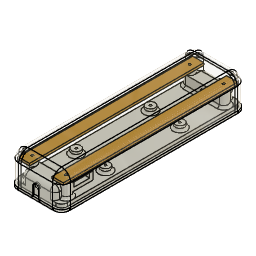
MQTT_Lamp (Autodesk Fusion 360 design; units mm, degrees)
Autodesk Fusion 360 part; units mm, degrees
sketch "Sketch1" plane through (0, 0, 0) normal (0, 0, 1) x (1, 0, 0) in component "base"
  line L0 (0, 0) -> (42, 0)
  line L1 (42, 0) -> (42, 160)
  line L2 (42, 160) -> (0, 160)
  line L3 (0, 160) -> (0, 0)
  dimension "d1" = 42
  dimension "d2" = 160
  constraint horizontal L0
  constraint vertical L1
  constraint horizontal L2
  constraint vertical L3
  constraint coincident L0.start L3.end
  measures "d1" distance of L0.start L0.end
  measures "d2" distance of L0.start L2.end
extrude "Extrude1" add sketch "Sketch1" along normal blind 5 makes body 1 in component "base"
sketch "Sketch2" plane through (0, 0, 5) normal (0, 0, 1) x (-1, 0, 0) in component "base"
  line L0 (0, -160) -> (0, 0)
  line L1 (0, 0) -> (-42, 0)
  line L2 (-42, 0) -> (-42, -160)
  line L3 (-42, -160) -> (0, -160)
  line L4 (-21, -160) -> (-21, 0)
  line L5 (-36, -150) -> (-6, -150)
  line L6 (-6, -150) -> (-6, -10)
  line L7 (-6, -10) -> (-36, -10)
  line L8 (-36, -10) -> (-36, -150)
  line L9 (-36, -150) -> (-6, -10) construction
  line L10 (-6, -150) -> (-36, -10) construction
  circle A0 centre (-6, -150) radius 1
  circle A1 centre (-36, -150) radius 1
  circle A2 centre (-6, -10) radius 1
  circle A3 centre (-36, -10) radius 1
  circle A4 centre (-36, -150) radius 4
  circle A5 centre (-6, -150) radius 4
  circle A6 centre (-6, -10) radius 4
  circle A7 centre (-36, -10) radius 4
  point P0 (-21, -80)
  dimension "d5" = 30
  dimension "d6" = 140
  dimension "d7" = 2
  dimension "d8" = 2
  dimension "d9" = 2
  dimension "d10" = 2
  dimension "d11" = 3
  dimension "d12" = 3
  dimension "d13" = 3
  dimension "d14" = 3
  constraint midpoint L3 L4.start
  constraint midpoint L1 L4.end
  constraint horizontal L5
  constraint perpendicular L5 L6
  constraint parallel L5 L7
  constraint parallel L6 L8
  constraint coincident L9 P0
  constraint coincident L10 P0
  constraint midpoint L4 P0
  constraint coincident L5.end L6.start
  constraint coincident L5.start L8.end
  constraint coincident L6.end L7.start
  constraint coincident L7.end L8.start
  measures "d5" distance of L6.end L7.end
  measures "d6" distance of L5.end L6.end
  measures "d7" diameter of A0
  measures "d8" diameter of A1
  measures "d9" diameter of A2
  measures "d10" diameter of A3
extrude "Extrude2" add sketch "Sketch2" along normal blind 14 contours L5 L8 A1 A4 | L5 L8 A1 A4 | L5 L6 A0 A5 | L5 L6 A0 A5 | L6 L7 A2 A6 | L6 L7 A2 A6 | L7 L8 A3 A7 | L7 L8 A3 A7 bodies 1 in component "base"
sketch "Sketch3" plane through (0, 0, 5) normal (0, 0, 1) x (-1, 0, 0) in component "base"
  circle A0 centre (-6, -150) radius 4
  circle A1 centre (-36, -150) radius 4
  line L0 (0, -160) -> (0, 0)
  line L1 (0, 0) -> (-42, 0)
  line L2 (-42, 0) -> (-42, -160)
  line L3 (-42, -160) -> (0, -160)
  circle A2 centre (-36, -10) radius 4
  circle A3 centre (-6, -10) radius 4
  line L4 (-6, -10) -> (-6, 0)
  line L5 (-6, 0) -> (-36, 0)
  line L6 (-36, 0) -> (-36, -14)
  line L7 (-36, -14) -> (-6, -14)
  line L8 (-6, -14) -> (-6, 0)
  line L9 (-36, -150) -> (-36, -160)
  line L10 (-36, -160) -> (-6, -160)
  line L11 (-6, -160) -> (-6, -146)
  line L12 (-6, -146) -> (-36, -146)
  line L13 (-36, -146) -> (-36, -160)
  constraint coincident A3.centre L4.start
  constraint coincident L1 L4.end
  constraint perpendicular L1 L4
  constraint horizontal L5
  constraint vertical L6
  constraint horizontal L7
  constraint vertical L8
  constraint coincident A2 L6.end
  constraint coincident A1.centre L9.start
  constraint coincident L3 L9.end
  constraint perpendicular L3 L9
  constraint horizontal L10
  constraint vertical L11
  constraint horizontal L12
  constraint vertical L13
  constraint coincident A0 L11.end
extrude "Extrude3" add sketch "Sketch3" along normal blind 10 contours A0 A1 L3 L9 L10 L11 L12 L13 | L1 A2 A3 L4 L5 L6 L7 L8 bodies 1 in component "base"
sketch "Sketch4" plane through (0, 0, 0) normal (0, -1, 0) x (1, 0, 0) in component "base"
  line L0 (0, 0) -> (42, 0)
  line L1 (42, 0) -> (42, 5)
  line L2 (42, 5) -> (36, 5)
  line L3 (36, 5) -> (36, 15)
  line L4 (36, 15) -> (6, 15)
  line L5 (6, 15) -> (6, 5)
  line L6 (6, 5) -> (0, 5)
  line L7 (0, 5) -> (0, 0)
  line L8 (6, 5) -> (36, 5)
  line L9 (21, 5) -> (21, 15)
  circle A0 centre (21, 10) radius 2.5
  dimension "d19" = 5
  constraint coincident L5.end L6.start
  constraint coincident L2.end L3.start
  constraint midpoint L8 L9.start
  constraint midpoint L4 L9.end
  constraint midpoint L9 A0.centre
  measures "d19" diameter of A0
extrude "Extrude4" cut sketch "Sketch4" against normal blind 14 contours L9 A0 | L9 A0 bodies 1 in component "base"
sketch "Sketch5" plane through (0, 160, 0) normal (0, 1, 0) x (-1, 0, 0) in component "base"
  line L0 (-42, 0) -> (0, 0)
  line L1 (0, 0) -> (0, 5)
  line L2 (0, 5) -> (-6, 5)
  line L3 (-6, 5) -> (-6, 15)
  line L4 (-6, 15) -> (-36, 15)
  line L5 (-36, 15) -> (-36, 5)
  line L6 (-36, 5) -> (-42, 5)
  line L7 (-42, 5) -> (-42, 0)
  line L8 (-36, 5) -> (-6, 5)
  line L9 (-21, 5) -> (-21, 15)
  circle A0 centre (-21, 10) radius 1.5
  dimension "d22" = 3
  constraint coincident L5.end L6.start
  constraint coincident L2.end L3.start
  constraint midpoint L8 L9.start
  constraint midpoint L4 L9.end
  constraint midpoint L9 A0.centre
  measures "d22" diameter of A0
extrude "Extrude5" cut sketch "Sketch5" against normal blind 14 contours L9 A0 | L9 A0 bodies 1 in component "base"
sketch "Sketch6" plane through (0, 0, 5) normal (0, 0, 1) x (-1, 0, 0) in component "base"
  line L0 (-6, -14) -> (-36, -14)
  arc A0 (-36, -6) -> (-36, -14) centre (-36, -10) ccw
  line L1 (-36, -6) -> (-36, 0)
  line L2 (-36, 0) -> (-42, 0)
  line L3 (-42, 0) -> (-42, -160)
  line L4 (-42, -160) -> (-36, -160)
  line L5 (-36, -160) -> (-36, -154)
  arc A1 (-36, -146) -> (-36, -154) centre (-36, -150) ccw
  line L6 (-36, -146) -> (-6, -146)
  arc A2 (-6, -154) -> (-6, -146) centre (-6, -150) ccw
  line L7 (-6, -154) -> (-6, -160)
  line L8 (-6, -160) -> (0, -160)
  line L9 (0, -160) -> (0, 0)
  line L10 (0, 0) -> (-6, 0)
  line L11 (-6, 0) -> (-6, -6)
  arc A3 (-6, -14) -> (-6, -6) centre (-6, -10) ccw
  line L12 (-36, -14) -> (-28, -14)
  line L13 (-28, -14) -> (-28, -34)
  line L14 (-28, -34) -> (-36, -34)
  line L15 (-36, -34) -> (-36, -14)
  dimension "d25" = 8
  dimension "d26" = 20
  constraint horizontal L12
  constraint vertical L13
  constraint horizontal L14
  constraint vertical L15
  constraint coincident L0.end A0.end
  measures "d25" distance of L0.end L12.end
  measures "d26" distance of L0.end L14.end
extrude "Extrude6" add sketch "Sketch6" along normal blind 10 contours L0 L12 L13 L14 L15 bodies 1 in component "base"
sketch "Sketch7" plane through (28, 0, 0) normal (-1, 0, 0) x (0, -1, 0) in component "base"
  line L0 (-34, 5) -> (-14, 5)
  line L1 (-14, 5) -> (-14, 15)
  line L2 (-14, 15) -> (-34, 15)
  line L3 (-34, 15) -> (-34, 5)
  line L4 (-31, 8) -> (-17, 8)
  line L5 (-17, 8) -> (-17, 12)
  line L6 (-17, 12) -> (-31, 12)
  line L7 (-31, 12) -> (-31, 8)
  dimension "d29" = -3
extrude "Extrude7" cut sketch "Sketch7" against normal blind 8 contours L4 L5 L6 L7 bodies 1 in component "base"
fillet "Fillet1" radius 3 2 edges at (28, 24, 15) (36, 24, 15) on bodies 1 in component "base"
fillet "Fillet2" radius 3 2 edges at (28.8787, 14, 14.1213) (28, 14, 8.5) on bodies 1 in component "base"
fillet "Fillet3" radius 5 4 edges at (42, 0, 2.5) (0, 0, 2.5) (42, 160, 2.5) (0, 160, 2.5) on bodies 1 in component "base"
fillet "Fillet4" radius 2 8 edges at (40, 150, 5) (21, 146, 5) (2, 150, 5) (40, 10, 5) (2, 10, 5) (15.5, 14, 5) (27.1213, 14.8787, 5) (28, 25.5, 5) on bodies 1 in component "base"
fillet "Fillet5" radius 4 10 edges at (6, 3, 15) (6, 0, 10) (21, 0, 15) (36, 0, 10) (36, 3, 15) (21, 160, 15) (36, 157, 15) (36, 160, 10) (6, 157, 15) (6, 160, 10) on bodies 1 in component "base"
sketch "Sketch9" plane through (0, 0, 5) normal (0, 0, 1) x (-1, 0, 0) in component "base"
  line L0 (-26, -34) -> (-36, -34)
  line L1 (-36, -34) -> (-36, -16)
  arc A0 (-42, -10) -> (-36, -16) centre (-36, -10) ccw
  line L2 (-42, -10) -> (-42, -150)
  arc A1 (-36, -144) -> (-42, -150) centre (-36, -150) ccw
  line L3 (-36, -144) -> (-6, -144)
  arc A2 (0, -150) -> (-6, -144) centre (-6, -150) ccw
  line L4 (0, -150) -> (0, -10)
  arc A3 (-6, -16) -> (0, -10) centre (-6, -10) ccw
  line L5 (-6, -16) -> (-25, -16)
  arc A4 (-25, -16) -> (-26, -17) centre (-25, -17) ccw
  line L6 (-26, -17) -> (-26, -34)
  line L7 (-42, -80) -> (0, -80)
  line L8 (-34, -113) -> (-8, -113)
  line L9 (-8, -113) -> (-8, -47)
  line L10 (-8, -47) -> (-34, -47)
  line L11 (-34, -47) -> (-34, -113)
  line L12 (-34, -113) -> (-8, -47) construction
  line L13 (-8, -113) -> (-34, -47) construction
  circle A5 centre (-8, -47) radius 1
  circle A6 centre (-34, -47) radius 1
  circle A7 centre (-8, -113) radius 1
  circle A8 centre (-34, -113) radius 1
  circle A9 centre (-34, -113) radius 4
  circle A10 centre (-8, -113) radius 4
  circle A11 centre (-8, -47) radius 4
  circle A12 centre (-34, -47) radius 4
  point P0 (-21, -80)
  dimension "d48" = 26
  dimension "d49" = 66
  dimension "d50" = 2
  dimension "d51" = 2
  dimension "d52" = 2
  dimension "d53" = 2
  dimension "d54" = 3
  dimension "d55" = 3
  dimension "d56" = 3
  dimension "d57" = 3
  constraint midpoint L2 L7.start
  constraint midpoint L4 L7.end
  constraint horizontal L8
  constraint perpendicular L8 L9
  constraint parallel L8 L10
  constraint parallel L9 L11
  constraint coincident L12 P0
  constraint coincident L13 P0
  constraint midpoint L7 P0
  constraint coincident L9.end L10.start
  constraint coincident L10.end L11.start
  constraint coincident L8.end L9.start
  constraint coincident L8.start L11.end
  measures "d48" distance of L9.end L10.end
  measures "d49" distance of L8.end L9.end
  measures "d50" diameter of A5
  measures "d51" diameter of A6
  measures "d52" diameter of A7
  measures "d53" diameter of A8
extrude "Extrude9" add sketch "Sketch9" along normal blind 4 contours L10 L11 A6 A12 | L10 L11 A6 A12 | L8 L11 A8 A9 | L8 L11 A8 A9 | L8 L9 A7 A10 | L8 L9 A7 A10 | L9 L10 A5 A11 | L9 L10 A5 A11 bodies 1 in component "base"
sketch "Sketch1 (2)" plane through (0, 0, 19) normal (0, 0, 1) x (-1, 0, 0) in component "light"
  circle A0 centre (-6, -10) radius 1
  circle A1 centre (-6, -10) radius 4
sketch "Sketch2 (2)" plane through (0, 0, 0) normal (0, 0, 1) x (1, 0, 0) in component "light"
  line L0 (0, 0) -> (10, 0)
  line L1 (10, 0) -> (10, 155)
  line L2 (10, 155) -> (0, 155)
  line L3 (0, 155) -> (0, 0)
  line L4 (5, 155) -> (5, 0)
  line L5 (5, 77.5) -> (5, 147.5)
  line L6 (5, 77.5) -> (5, 7.5)
  circle A0 centre (5, 7.5) radius 1
  circle A1 centre (5, 147.5) radius 1
  dimension "d62" = 10
  dimension "d63" = 155
  dimension "d64" = 70
  dimension "d65" = 70
  dimension "d66" = 2
  dimension "d67" = 2
  constraint horizontal L0
  constraint vertical L1
  constraint horizontal L2
  constraint vertical L3
  constraint coincident L0.start L3.end
  constraint midpoint L2 L4.start
  constraint midpoint L0 L4.end
  constraint midpoint L4 L5.start
  constraint perpendicular L0 L5
  constraint parallel L4 L6
  constraint coincident L6.end A0.centre
  constraint coincident L5.end A1.centre
  measures "d62" distance of L0.start L0.end
  measures "d63" distance of L0.start L2.end
  measures "d64" distance of L5.start L5.end
  measures "d65" distance of L5.start L6.end
  measures "d66" diameter of A0
  measures "d67" diameter of A1
extrude "Extrude1'" add sketch "Sketch2 (2)" along normal blind 2 separate body contours L0 L2 L3 L4 L5 L6 A0 A1 | L0 L1 L2 L4 L5 L6 A0 A1 makes body 2 in component "light"
move_body "Move1" bodies 2 to x (1, 0, 0) y (0, 1, 0) z (0, 0, 1) at (1, 2.5, 19) in component "light"
sketch "Sketch1 (3)" plane through (0, 0, 0) normal (0, 0, -1) x (1, 0, 0)
  arc A0 (0, -155) -> (5, -160) centre (5, -155) ccw
  line L0 (5, -160) -> (37, -160)
  arc A1 (37, -160) -> (42, -155) centre (37, -155) ccw
  line L1 (42, -155) -> (42, -5)
  arc A2 (42, -5) -> (37, 0) centre (37, -5) ccw
  line L2 (37, 0) -> (5, 0)
  arc A3 (5, 0) -> (0, -5) centre (5, -5) ccw
  line L3 (0, -5) -> (0, -155)
  line L4 (37, 2) -> (5, 2)
  arc A4 (5, 2) -> (-2, -5) centre (5, -5) ccw
  line L5 (-2, -5) -> (-2, -155)
  arc A5 (-2, -155) -> (5, -162) centre (5, -155) ccw
  line L6 (5, -162) -> (37, -162)
  arc A6 (37, -162) -> (44, -155) centre (37, -155) ccw
  line L7 (44, -155) -> (44, -5)
  arc A7 (44, -5) -> (37, 2) centre (37, -5) ccw
  dimension "d70" = 2
extrude "Extrude10" add sketch "Sketch1 (3)" against normal blind 2 bodies 1 in component "base"
sketch "Sketch2 (3)" plane through (0, 0, 5) normal (0, 0, 1) x (-1, 0, 0)
  line L0 (-26, -34) -> (-36, -34)
  line L1 (-36, -34) -> (-36, -16)
  arc A0 (-42, -10) -> (-36, -16) centre (-36, -10) ccw
  line L2 (-42, -10) -> (-42, -150)
  arc A1 (-36, -144) -> (-42, -150) centre (-36, -150) ccw
  line L3 (-36, -144) -> (-6, -144)
  arc A2 (0, -150) -> (-6, -144) centre (-6, -150) ccw
  line L4 (0, -150) -> (0, -10)
  arc A3 (-6, -16) -> (0, -10) centre (-6, -10) ccw
  line L5 (-6, -16) -> (-25, -16)
  arc A4 (-25, -16) -> (-26, -17) centre (-25, -17) ccw
  line L6 (-26, -17) -> (-26, -34)
  line L7 (-21, -144) -> (-21, -16)
  line L8 (-21, -80) -> (-21, -130)
  line L9 (-21, -80) -> (-21, -30)
  circle A5 centre (-21, -30) radius 2
  circle A6 centre (-21, -130) radius 2
  circle A7 centre (-8, -47) radius 4
  circle A8 centre (-34, -47) radius 4
  circle A9 centre (-34, -113) radius 4
  circle A10 centre (-8, -113) radius 4
  dimension "d73" = 50
  dimension "d74" = 4
  dimension "d75" = 4
  constraint midpoint L3 L7.start
  constraint coincident L5 L7.end
  constraint perpendicular L5 L7
  constraint midpoint L7 L8.start
  constraint coincident L7 L8.end
  constraint parallel L7 L9
  constraint coincident L9.end A5.centre
  constraint coincident L8.end A6.centre
  measures "d73" distance of L8.start L9.end
  measures "d74" diameter of A5
  measures "d75" diameter of A6
extrude "Extrude11" cut sketch "Sketch2 (3)" against normal blind 5 contours L7 L9 A5 | L7 L9 A5 | L7 L8 A6 | L7 L8 A6 bodies 1 in component "base"
extrude "Extrude12" cut 4 faces at (8.2754, 47.2871, 5) (8.226, 113.5035, 5) (33.8333, 113.388, 5) (34.2078, 47.36, 5) along direction (0, 0, -1) blind 5 on bodies 1 bodies 1 in component "base"
sketch "Sketch3 (2)" plane through (0, 0, 5) normal (0, 0, 1) x (-1, 0, 0)
  circle A0 centre (-21, -130) radius 2
  circle A1 centre (-21, -30) radius 2
  circle A2 centre (-8, -47) radius 4
  circle A3 centre (-34, -47) radius 4
  line L0 (-26, -34) -> (-36, -34)
  line L1 (-36, -34) -> (-36, -16)
  arc A4 (-42, -10) -> (-36, -16) centre (-36, -10) ccw
  line L2 (-42, -10) -> (-42, -150)
  arc A5 (-36, -144) -> (-42, -150) centre (-36, -150) ccw
  line L3 (-36, -144) -> (-6, -144)
  arc A6 (0, -150) -> (-6, -144) centre (-6, -150) ccw
  line L4 (0, -150) -> (0, -10)
  arc A7 (-6, -16) -> (0, -10) centre (-6, -10) ccw
  line L5 (-6, -16) -> (-25, -16)
  arc A8 (-25, -16) -> (-26, -17) centre (-25, -17) ccw
  line L6 (-26, -17) -> (-26, -34)
  circle A9 centre (-34, -113) radius 4
  circle A10 centre (-8, -113) radius 4
fillet "Fillet7" radius 2 4 edges at (11.7293, 45.5535, 5) (37.7293, 45.5535, 5) (37.7293, 111.5535, 5) (11.7293, 111.5535, 5) on bodies 1 in component "base"
sketch "Sketch1 (4)" plane through (0, 0, 5) normal (0, 0, 1) x (-1, 0, 0) in component "hood"
sketch "Sketch2 (4)" plane through (0, 0, 0) normal (0, 0, 1) x (1, 0, 0) in component "hood"
sketch "Sketch3 (3)" plane through (0, 0, 0) normal (0, 0, 1) x (1, 0, 0) in component "hood"
  line L0 (0, 0) -> (42, 0)
  line L1 (42, 0) -> (42, 160)
  line L2 (42, 160) -> (0, 160)
  line L3 (0, 160) -> (0, 0)
  line L4 (44, 162) -> (-2, 162)
  line L5 (-2, 162) -> (-2, -2)
  line L6 (-2, -2) -> (44, -2)
  line L7 (44, -2) -> (44, 162)
  line L8 (43, 161) -> (-1, 161)
  line L9 (-1, 161) -> (-1, -1)
  line L10 (-1, -1) -> (43, -1)
  line L11 (43, -1) -> (43, 161)
  dimension "d82" = 2
  dimension "d83" = 1
  constraint horizontal L0
  constraint vertical L1
  constraint horizontal L2
  constraint vertical L3
  constraint coincident L0.start L3.end
extrude "Extrude1''" add sketch "Sketch3 (3)" along normal blind 21 separate body contours L4 L5 L6 L7 makes body 3 in component "hood"
extrude "Extrude2'" add 1 faces at (-1.6667, 53, 21) along direction (0, 0, 1) blind 8 on bodies 3 bodies 3 in component "hood"
sketch "Sketch4 (2)" plane through (-1, 0, 0) normal (1, 0, 0) x (0, 1, 0) in component "hood"
  line L0 (-1, 0) -> (161, 0)
  line L1 (161, 0) -> (161, 29)
  line L2 (161, 29) -> (-1, 29)
  line L3 (-1, 29) -> (-1, 0)
  line L4 (-1, 29) -> (-1, 28)
  line L5 (-1, 28) -> (161, 28)
  line L6 (161, 28) -> (161, 29)
  line L7 (161, 29) -> (-1, 29)
  line L8 (-1, 29) -> (-1, 28)
  dimension "d88" = 1
  constraint coincident L2.end L3.start
  constraint perpendicular L2 L4
  constraint horizontal L5
  constraint vertical L6
  constraint horizontal L7
  constraint vertical L8
  constraint coincident L1.end L2.start
  measures "d88" distance of L2.end L4.end
extrude "Extrude3'" add sketch "Sketch4 (2)" along normal blind 44 contours L1 L2 L3 L4 L5 L6 L7 L8 bodies 3 in component "hood"
fillet "Fillet1'" radius 8 8 edges at (21, 161, 28) (43, 80, 28) (21, -1, 28) (-1, 80, 28) (-2, 80, 29) (21, -2, 29) (44, 80, 29) (21, 162, 29) on bodies 3 in component "hood"
fillet "Fillet2'" radius 8 16 edges at (-2, -2, 10.5) (0.3431, 0.3431, 26.6569) (44, -2, 10.5) (41.6569, 0.3431, 26.6569) (-2, 162, 10.5) (0.3431, 159.6569, 26.6569) (44, 162, 10.5) (41.6569, 159.6569, 26.6569) (43, 161, 10) (40.6569, 158.6569, 25.6569) (-1, 161, 10) (1.3431, 158.6569, 25.6569) (-1, -1, 10) (1.3431, 1.3431, 25.6569) (43, -1, 10) (40.6569, 1.3431, 25.6569) on bodies 3 in component "hood"
sketch "Sketch10" plane through (0, 0, 0) normal (0, -1, 0) x (1, 0, 0) in component "base"
  line L0 (5, 2) -> (37, 2)
  line L1 (37, 2) -> (37, 5)
  line L2 (37, 5) -> (32, 5)
  line L3 (32, 5) -> (32, 11)
  line L4 (32, 11) -> (23.2913, 11)
  arc A0 (18.7087, 11) -> (23.2913, 11) centre (21, 10) ccw
  line L5 (18.7087, 11) -> (10, 11)
  line L6 (10, 11) -> (10, 5)
  line L7 (10, 5) -> (5, 5)
  line L8 (5, 5) -> (5, 2)
  circle A1 centre (21, 10) radius 2.5
  constraint concentric A0 A1
extrude "Extrude4'" cut sketch "Sketch10" along normal blind 19 contours A0 A1 bodies 3 in component "hood"
sketch "Sketch11" plane through (0, 160, 0) normal (0, 1, 0) x (-1, 0, 0) in component "base"
  line L0 (-37, 2) -> (-5, 2)
  line L1 (-5, 2) -> (-5, 5)
  line L2 (-5, 5) -> (-10, 5)
  line L3 (-10, 5) -> (-10, 11)
  line L4 (-10, 11) -> (-19.882, 11)
  arc A0 (-22.118, 11) -> (-19.882, 11) centre (-21, 10) ccw
  line L5 (-22.118, 11) -> (-32, 11)
  line L6 (-32, 11) -> (-32, 5)
  line L7 (-32, 5) -> (-37, 5)
  line L8 (-37, 5) -> (-37, 2)
  circle A1 centre (-21, 10) radius 1.5
  constraint concentric A0 A1
extrude "Extrude5'" cut sketch "Sketch11" along normal blind 19 contours A0 A1 bodies 3 in component "hood"
sketch "Sketch5 (2)" plane through (0, -2, 0) normal (0, -1, 0) x (1, 0, 0) in component "hood"
  circle A0 centre (21, 10) radius 2.5
  line L0 (36, 0) -> (36, 21)
  line L1 (36, 21) -> (6, 21)
  line L2 (6, 21) -> (6, 0)
  line L3 (6, 0) -> (36, 0)
  line L4 (23.5, 10) -> (23.5, 0)
  line L5 (18.5, 10) -> (18.5, 0)
  circle A1 centre (21, 10) radius 2.5
  constraint coincident A0 L4.start
  constraint coincident L3 L4.end
  constraint tangent A0 L4
  constraint perpendicular L3 L4
  constraint coincident A0 L5.start
  constraint coincident L3 L5.end
  constraint tangent A0 L5
  constraint perpendicular L3 L5
  constraint concentric A0 A1
  constraint coincident L4.start A1
extrude "Extrude6'" cut sketch "Sketch5 (2)" against normal blind 1 contours A0 L3 L4 L5 A1 bodies 3 in component "hood"
fillet "Fillet3'" radius 3 2 edges at (23.5, -1.5, 0) (18.5, -1.5, 0) on bodies 3 in component "hood"
component "base" placed x (1, 0, 0) y (0, 1, 0) z (0, 0, 1) at (0, 0, 0)
component "light" placed x (1, 0, 0) y (0, 1, 0) z (0, 0, 1) at (0, 0, 0)
component "light" placed x (1, 0, 0) y (0, 1, 0) z (0, 0, 1) at (30, 0, 0)
component "hood" placed x (1, 0, 0) y (0, 1, 0) z (0, 0, 1) at (0, 0, 0)
